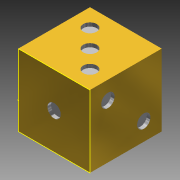
# Autodesk Inventor part: Part7
Saved by Autodesk Inventor 2013 (Build 170138000, 138)
## iProperties
Created: 2013-08-29
Part Number: Part7
Material: Generic
Document SubType Name: Modeling
Designer: s601298
Density: 1 g/cm^3
Author: s601298
Autodesk Inventor part; units mm, degrees
ref_plane "YZ Plane" through (0, 0, 0) normal (1, 0, 0) x (0, 1, 0)
ref_plane "XZ Plane" through (0, 0, 0) normal (0, 1, 0) x (-1, 0, 0)
ref_plane "XY Plane" through (0, 0, 0) normal (0, 0, 1) x (1, 0, 0)
sketch "Sketch1" plane through (0, 0, 0) normal (1, 0, 0) x (0, 1, 0)
  line L0 (15.7193, -14.4333) -> (-9.6807, -14.4333)
  line L1 (-9.6807, -14.4333) -> (-9.6807, 10.9667)
  line L2 (-9.6807, 10.9667) -> (15.7193, 10.9667)
  line L3 (15.7193, 10.9667) -> (15.7193, -14.4333)
  line L4 (15.7193, -14.4333) -> (-9.6807, 10.9667) construction
  line L5 (-9.6807, -14.4333) -> (15.7193, 10.9667) construction
  point P0 (0, 0)
  point P1 (3.0193, -1.7333)
  dimension "d0" = 25.4
  dimension "d1" = 25.4
  constraints: 12 end point, 2 midpoint, 2 parallel, 1 horizontal, 1 perpendicular
  measures "d0" distance of L1.end L2.end
  measures "d1" distance of L0.end L1.end
extrude "Extrusion1" add sketch "Sketch1" along normal blind 25.4
sketch "Sketch2" plane through (0, -9.6807, 10.9667) normal (0, 0, 1) x (1, 0, 0)
  circle A0 centre (12.7, 12.7) radius 2.3749
  point P0 (0, 9.6807)
  dimension "d4" = 4.7498
  constraints: 1 centre point
  measures "d4" diameter of A0
sketch "Sketch3" plane through (0, -9.6807, 10.9667) normal (0, 0, 1) x (1, 0, 0)
  line L0 (0, 0) -> (0, 25.4) projected
  line L1 (0, 0) -> (25.4, 0) projected
  line L2 (25.4, 25.4) -> (25.4, 0) projected
  line L3 (0, 25.4) -> (25.4, 25.4) projected
  point P0 (0, 9.6807)
extrude "Extrusion2" cut sketch "Sketch2" against normal blind 1.27
sketch "Sketch4" plane through (0, 15.7193, 10.9667) normal (0, 1, 0) x (1, 0, 0)
  circle A0 centre (6.3453, 19.0547) radius 2.3749
  circle A1 centre (12.7, 12.7) radius 2.3749
  circle A2 centre (19.0547, 6.3453) radius 2.3749
  point P0 (0, 10.9667)
  dimension "d7" = 4.7498
  dimension "d8" = 4.7498
  dimension "d9" = 4.7498
  constraints: 3 centre point
  measures "d7" diameter of A0
  measures "d8" diameter of A1
  measures "d9" diameter of A2
extrude "Extrusion3" cut sketch "Sketch4" against normal blind 1.27
sketch "Sketch5" plane through (0, -9.6807, -14.4333) normal (0, -1, 0) x (1, 0, 0)
  circle A0 centre (6.3453, 19.0547) radius 2.3749
  circle A1 centre (19.0547, 19.0547) radius 2.3749
  circle A2 centre (6.3453, 6.3453) radius 2.3749
  circle A3 centre (19.0547, 6.3453) radius 2.3749
  point P0 (0, 14.4333)
  dimension "d12" = 4.7498
  dimension "d13" = 4.7498
  dimension "d14" = 4.7498
  dimension "d15" = 4.7498
  constraints: 4 centre point
  measures "d12" diameter of A0
  measures "d13" diameter of A1
  measures "d14" diameter of A2
  measures "d15" diameter of A3
extrude "Extrusion4" cut sketch "Sketch5" against normal blind 1.27
sketch "Sketch6" plane through (0, -9.6807, -14.4333) normal (0, 0, -1) x (-1, 0, 0)
  circle A0 centre (-19.0556, 19.0556) radius 2.3749
  circle A1 centre (-6.3444, 19.0556) radius 2.3749
  circle A2 centre (-6.3444, 6.3444) radius 2.3749
  circle A3 centre (-19.0556, 6.3444) radius 2.3749
  circle A4 centre (-6.3444, 12.7) radius 2.3749
  circle A5 centre (-19.0556, 12.7) radius 2.3749
  point P0 (0, 9.6807)
  dimension "d18" = 4.7498
  dimension "d19" = 4.7498
  dimension "d20" = 4.7498
  dimension "d21" = 4.7498
  dimension "d22" = 4.7498
  dimension "d23" = 4.7498
  constraints: 6 centre point
  measures "d18" diameter of A0
  measures "d19" diameter of A1
  measures "d20" diameter of A2
  measures "d21" diameter of A3
  measures "d22" diameter of A4
  measures "d23" diameter of A5
extrude "Extrusion5" cut sketch "Sketch6" against normal blind 1.27
sketch "Sketch7" plane through (0, 0, 0) normal (-1, 0, 0) x (0, 0, 1)
  line L0 (-14.4333, 15.7193) -> (-14.4333, -9.6807) projected
  line L1 (-14.4333, -9.6807) -> (10.9667, -9.6807) projected
  line L2 (10.9667, -9.6807) -> (10.9667, 15.7193) projected
  line L3 (10.9667, 15.7193) -> (-14.4333, 15.7193) projected
  circle A0 centre (-8.0833, 9.3693) radius 2.3749
  circle A1 centre (4.6222, 9.3693) radius 2.3749
  circle A2 centre (4.6222, -3.3307) radius 2.3749
  circle A3 centre (-8.0833, -3.3307) radius 2.3749
  circle A4 centre (-1.7333, 3.0193) radius 2.3749
  point P0 (0, 0)
  dimension "d26" = 6.35
  dimension "d27" = 6.35
  dimension "d28" = 6.35
  dimension "d29" = 6.3444
  dimension "d30" = 6.35
  dimension "d31" = 6.3444
  dimension "d32" = 6.35
  dimension "d33" = 6.35
  dimension "d34" = 12.7
  dimension "d35" = 12.7
  dimension "d36" = 4.7498
  dimension "d37" = 4.7498
  dimension "d38" = 4.7498
  dimension "d39" = 4.7498
  dimension "d40" = 4.7498
  constraints: 5 centre point
  measures "d26" distance from line of A0.centre L3
  measures "d27" distance from line of A0.centre L0
  measures "d28" distance from line of A1.centre L3
  measures "d29" distance from line of A1.centre L2
  measures "d30" distance from line of A2.centre L1
  measures "d31" distance from line of A2.centre L2
  measures "d32" distance from line of A3.centre L0
  measures "d33" distance from line of A3.centre L1
  measures "d34" distance from line of A4.centre L2
  measures "d35" distance from line of A4.centre L3
  measures "d36" diameter of A0
  measures "d37" diameter of A1
  measures "d38" diameter of A4
  measures "d39" diameter of A3
  measures "d40" diameter of A2
extrude "Extrusion6" cut sketch "Sketch7" against normal blind 1.27 contours A0 | A1 | A2 | A3 | A4
sketch "Sketch8" plane through (25.4, 0, 0) normal (1, 0, 0) x (0, 0, -1)
  line L0 (14.4333, -9.6807) -> (14.4333, 15.7193) projected
  line L1 (14.4333, 15.7193) -> (-10.9667, 15.7193) projected
  line L2 (-10.9667, 15.7193) -> (-10.9667, -9.6807) projected
  line L3 (-10.9667, -9.6807) -> (14.4333, -9.6807) projected
  circle A0 centre (-4.6167, 9.3693) radius 2.3749
  circle A1 centre (8.0833, -3.3307) radius 2.3749
  point P0 (0, 0)
  dimension "d43" = 4.7498
  dimension "d44" = 4.7498
  dimension "d45" = 6.35
  dimension "d46" = 6.35
  dimension "d47" = 6.35
  dimension "d48" = 6.35
  constraints: 2 centre point
  measures "d43" diameter of A0
  measures "d44" diameter of A1
  measures "d45" distance from line of A0.centre L1
  measures "d46" distance from line of A0.centre L2
  measures "d47" distance from line of A1.centre L0
  measures "d48" distance from line of A1.centre L3
extrude "Extrusion7" cut sketch "Sketch8" against normal blind 1.27 contours A0 | A1
body "Solid1"
